Autodesk Fusion 360 part; units mm, degrees
(part 2 of 3)
  arc A308 (601.5, 1) -> (601, 0.5) centre (601.5, 0.5) ccw
  arc A309 (605, 0.5) -> (604.5, 1) centre (604.5, 0.5) ccw
  arc A310 (604.5, -3) -> (605, -2.5) centre (604.5, -2.5) ccw
  arc A311 (601, -2.5) -> (601.5, -3) centre (601.5, -2.5) ccw
  arc A312 (606.5, 1) -> (606, 0.5) centre (606.5, 0.5) ccw
  arc A313 (610, 0.5) -> (609.5, 1) centre (609.5, 0.5) ccw
  arc A314 (609.5, -3) -> (610, -2.5) centre (609.5, -2.5) ccw
  arc A315 (606, -2.5) -> (606.5, -3) centre (606.5, -2.5) ccw
  arc A316 (611.5, 1) -> (611, 0.5) centre (611.5, 0.5) ccw
  arc A317 (615, 0.5) -> (614.5, 1) centre (614.5, 0.5) ccw
  arc A318 (611, -2.5) -> (611.5, -3) centre (611.5, -2.5) ccw
  arc A319 (614.5, -3) -> (615, -2.5) centre (614.5, -2.5) ccw
  arc A320 (616.5, 1) -> (616, 0.5) centre (616.5, 0.5) ccw
  arc A321 (620, 0.5) -> (619.5, 1) centre (619.5, 0.5) ccw
  arc A322 (619.5, -3) -> (620, -2.5) centre (619.5, -2.5) ccw
  arc A323 (616, -2.5) -> (616.5, -3) centre (616.5, -2.5) ccw
  arc A324 (621, -2.5) -> (621.5, -3) centre (621.5, -2.5) ccw
  arc A325 (624.5, -3) -> (625, -2.5) centre (624.5, -2.5) ccw
  arc A326 (625, 0.5) -> (624.5, 1) centre (624.5, 0.5) ccw
  arc A327 (621.5, 1) -> (621, 0.5) centre (621.5, 0.5) ccw
  arc A328 (626.5, 1) -> (626, 0.5) centre (626.5, 0.5) ccw
  arc A329 (630, 0.5) -> (629.5, 1) centre (629.5, 0.5) ccw
  arc A330 (629.5, -3) -> (630, -2.5) centre (629.5, -2.5) ccw
  arc A331 (626, -2.5) -> (626.5, -3) centre (626.5, -2.5) ccw
  arc A332 (631, -2.5) -> (631.5, -3) centre (631.5, -2.5) ccw
  arc A333 (634.5, -3) -> (635, -2.5) centre (634.5, -2.5) ccw
  arc A334 (635, 0.5) -> (634.5, 1) centre (634.5, 0.5) ccw
  arc A335 (631.5, 1) -> (631, 0.5) centre (631.5, 0.5) ccw
  arc A336 (636.5, 1) -> (636, 0.5) centre (636.5, 0.5) ccw
  arc A337 (640, 0.5) -> (639.5, 1) centre (639.5, 0.5) ccw
  arc A338 (639.5, -3) -> (640, -2.5) centre (639.5, -2.5) ccw
  arc A339 (636, -2.5) -> (636.5, -3) centre (636.5, -2.5) ccw
  arc A340 (641.5, 1) -> (641, 0.5) centre (641.5, 0.5) ccw
  arc A341 (645, 0.5) -> (644.5, 1) centre (644.5, 0.5) ccw
  arc A342 (644.5, -3) -> (645, -2.5) centre (644.5, -2.5) ccw
  arc A343 (641, -2.5) -> (641.5, -3) centre (641.5, -2.5) ccw
  arc A344 (646.5, 1) -> (646, 0.5) centre (646.5, 0.5) ccw
  arc A345 (650, 0.5) -> (649.5, 1) centre (649.5, 0.5) ccw
  arc A346 (649.5, -3) -> (650, -2.5) centre (649.5, -2.5) ccw
  arc A347 (646, -2.5) -> (646.5, -3) centre (646.5, -2.5) ccw
  arc A348 (651.5, 1) -> (651, 0.5) centre (651.5, 0.5) ccw
  arc A349 (655, 0.5) -> (654.5, 1) centre (654.5, 0.5) ccw
  arc A350 (651, -2.5) -> (651.5, -3) centre (651.5, -2.5) ccw
  arc A351 (654.5, -3) -> (655, -2.5) centre (654.5, -2.5) ccw
  arc A352 (656.5, 1) -> (656, 0.5) centre (656.5, 0.5) ccw
  arc A353 (656, -2.5) -> (656.5, -3) centre (656.5, -2.5) ccw
  arc A354 (659.5, -3) -> (660, -2.5) centre (659.5, -2.5) ccw
  arc A355 (660, 0.5) -> (659.5, 1) centre (659.5, 0.5) ccw
  arc A356 (597.5, -4) -> (597, -4.5) centre (597.5, -4.5) ccw
  arc A357 (597, -7.5) -> (597.5, -8) centre (597.5, -7.5) ccw
  arc A358 (602.5, -8) -> (603, -7.5) centre (602.5, -7.5) ccw
  arc A359 (603, -4.5) -> (602.5, -4) centre (602.5, -4.5) ccw
  arc A360 (604.5, -4) -> (604, -4.5) centre (604.5, -4.5) ccw
  arc A361 (604, -7.5) -> (604.5, -8) centre (604.5, -7.5) ccw
  arc A362 (607.5, -8) -> (608, -7.5) centre (607.5, -7.5) ccw
  arc A363 (608, -4.5) -> (607.5, -4) centre (607.5, -4.5) ccw
  arc A364 (609.5, -4) -> (609, -4.5) centre (609.5, -4.5) ccw
  arc A365 (609, -7.5) -> (609.5, -8) centre (609.5, -7.5) ccw
  arc A366 (612.5, -8) -> (613, -7.5) centre (612.5, -7.5) ccw
  arc A367 (613, -4.5) -> (612.5, -4) centre (612.5, -4.5) ccw
  arc A368 (614.5, -4) -> (614, -4.5) centre (614.5, -4.5) ccw
  arc A369 (614, -7.5) -> (614.5, -8) centre (614.5, -7.5) ccw
  arc A370 (617.5, -8) -> (618, -7.5) centre (617.5, -7.5) ccw
  arc A371 (618, -4.5) -> (617.5, -4) centre (617.5, -4.5) ccw
  arc A372 (619.5, -4) -> (619, -4.5) centre (619.5, -4.5) ccw
  arc A373 (619, -7.5) -> (619.5, -8) centre (619.5, -7.5) ccw
  arc A374 (622.5, -8) -> (623, -7.5) centre (622.5, -7.5) ccw
  arc A375 (623, -4.5) -> (622.5, -4) centre (622.5, -4.5) ccw
  arc A376 (624.5, -4) -> (624, -4.5) centre (624.5, -4.5) ccw
  arc A377 (624, -7.5) -> (624.5, -8) centre (624.5, -7.5) ccw
  arc A378 (627.5, -8) -> (628, -7.5) centre (627.5, -7.5) ccw
  arc A379 (628, -4.5) -> (627.5, -4) centre (627.5, -4.5) ccw
  arc A380 (629.5, -4) -> (629, -4.5) centre (629.5, -4.5) ccw
  arc A381 (629, -7.5) -> (629.5, -8) centre (629.5, -7.5) ccw
  arc A382 (632.5, -8) -> (633, -7.5) centre (632.5, -7.5) ccw
  arc A383 (633, -4.5) -> (632.5, -4) centre (632.5, -4.5) ccw
  arc A384 (634.5, -4) -> (634, -4.5) centre (634.5, -4.5) ccw
  arc A385 (634, -7.5) -> (634.5, -8) centre (634.5, -7.5) ccw
  arc A386 (637.5, -8) -> (638, -7.5) centre (637.5, -7.5) ccw
  arc A387 (638, -4.5) -> (637.5, -4) centre (637.5, -4.5) ccw
  arc A388 (639.5, -4) -> (639, -4.5) centre (639.5, -4.5) ccw
  arc A389 (639, -7.5) -> (639.5, -8) centre (639.5, -7.5) ccw
  arc A390 (642.5, -8) -> (643, -7.5) centre (642.5, -7.5) ccw
  arc A391 (643, -4.5) -> (642.5, -4) centre (642.5, -4.5) ccw
  arc A392 (644.5, -4) -> (644, -4.5) centre (644.5, -4.5) ccw
  arc A393 (644, -7.5) -> (644.5, -8) centre (644.5, -7.5) ccw
  arc A394 (647.5, -8) -> (648, -7.5) centre (647.5, -7.5) ccw
  arc A395 (648, -4.5) -> (647.5, -4) centre (647.5, -4.5) ccw
  arc A396 (649.5, -4) -> (649, -4.5) centre (649.5, -4.5) ccw
  arc A397 (649, -7.5) -> (649.5, -8) centre (649.5, -7.5) ccw
  arc A398 (652.5, -8) -> (653, -7.5) centre (652.5, -7.5) ccw
  arc A399 (653, -4.5) -> (652.5, -4) centre (652.5, -4.5) ccw
  arc A400 (654.5, -4) -> (654, -4.5) centre (654.5, -4.5) ccw
  arc A401 (654, -7.5) -> (654.5, -8) centre (654.5, -7.5) ccw
  arc A402 (657.5, -8) -> (658, -7.5) centre (657.5, -7.5) ccw
  arc A403 (658, -4.5) -> (657.5, -4) centre (657.5, -4.5) ccw
  arc A404 (626, -12.5) -> (626.5, -13) centre (626.5, -12.5) ccw
  arc A405 (629.5, -13) -> (630, -12.5) centre (629.5, -12.5) ccw
  arc A406 (629, -14.5) -> (628.5, -14) centre (628.5, -14.5) ccw
  arc A407 (625.5, -14) -> (625, -14.5) centre (625.5, -14.5) ccw
  arc A408 (625, -17.5) -> (625.5, -18) centre (625.5, -17.5) ccw
  arc A409 (623.5, -18) -> (624, -17.5) centre (623.5, -17.5) ccw
  arc A410 (624, -14.5) -> (623.5, -14) centre (623.5, -14.5) ccw
  arc A411 (620.5, -14) -> (620, -14.5) centre (620.5, -14.5) ccw
  arc A412 (620, -17.5) -> (620.5, -18) centre (620.5, -17.5) ccw
  arc A413 (617.5, -19) -> (617, -19.5) centre (617.5, -19.5) ccw
  arc A414 (617, -22.5) -> (617.5, -23) centre (617.5, -22.5) ccw
  arc A415 (615.5, -23) -> (616, -22.5) centre (615.5, -22.5) ccw
  arc A416 (616, -19.5) -> (615.5, -19) centre (615.5, -19.5) ccw
  arc A417 (612.5, -19) -> (612, -19.5) centre (612.5, -19.5) ccw
  arc A418 (612, -22.5) -> (612.5, -23) centre (612.5, -22.5) ccw
  arc A419 (610.5, -23) -> (611, -22.5) centre (610.5, -22.5) ccw
  arc A420 (611, -19.5) -> (610.5, -19) centre (610.5, -19.5) ccw
  arc A421 (607.5, -19) -> (607, -19.5) centre (607.5, -19.5) ccw
  arc A422 (607, -22.5) -> (607.5, -23) centre (607.5, -22.5) ccw
  arc A423 (619, -14.5) -> (618.5, -14) centre (618.5, -14.5) ccw
  arc A424 (618.5, -18) -> (619, -17.5) centre (618.5, -17.5) ccw
  arc A425 (615, -17.5) -> (615.5, -18) centre (615.5, -17.5) ccw
  arc A426 (615.5, -14) -> (615, -14.5) centre (615.5, -14.5) ccw
  arc A427 (624.5, -13) -> (625, -12.5) centre (624.5, -12.5) ccw
  arc A428 (621.5, -9) -> (621, -9.5) centre (621.5, -9.5) ccw
  arc A429 (621, -12.5) -> (621.5, -13) centre (621.5, -12.5) ccw
  arc A430 (619.5, -13) -> (620, -12.5) centre (619.5, -12.5) ccw
  arc A431 (620, -9.5) -> (619.5, -9) centre (619.5, -9.5) ccw
  arc A432 (616.5, -9) -> (616, -9.5) centre (616.5, -9.5) ccw
  arc A433 (616, -12.5) -> (616.5, -13) centre (616.5, -12.5) ccw
  arc A434 (614.5, -13) -> (615, -12.5) centre (614.5, -12.5) ccw
  arc A435 (615, -9.5) -> (614.5, -9) centre (614.5, -9.5) ccw
  arc A436 (611.5, -9) -> (611, -9.5) centre (611.5, -9.5) ccw
  arc A437 (611, -12.5) -> (611.5, -13) centre (611.5, -12.5) ccw
  arc A438 (614, -14.5) -> (613.5, -14) centre (613.5, -14.5) ccw
  arc A439 (613.5, -18) -> (614, -17.5) centre (613.5, -17.5) ccw
  arc A440 (610, -17.5) -> (610.5, -18) centre (610.5, -17.5) ccw
  arc A441 (610.5, -14) -> (610, -14.5) centre (610.5, -14.5) ccw
  arc A442 (609.5, -13) -> (610, -12.5) centre (609.5, -12.5) ccw
  arc A443 (610, -9.5) -> (609.5, -9) centre (609.5, -9.5) ccw
  arc A444 (606.5, -9) -> (606, -9.5) centre (606.5, -9.5) ccw
  arc A445 (606, -12.5) -> (606.5, -13) centre (606.5, -12.5) ccw
  arc A446 (609, -14.5) -> (608.5, -14) centre (608.5, -14.5) ccw
  arc A447 (608.5, -18) -> (609, -17.5) centre (608.5, -17.5) ccw
  arc A448 (606, -19.5) -> (605.5, -19) centre (605.5, -19.5) ccw
  arc A449 (605.5, -23) -> (606, -22.5) centre (605.5, -22.5) ccw
  arc A450 (597.5, -9) -> (597, -9.5) centre (597.5, -9.5) ccw
  arc A451 (605, -9.5) -> (604.5, -9) centre (604.5, -9.5) ccw
  arc A452 (597, -12.5) -> (597.5, -13) centre (597.5, -12.5) ccw
  arc A453 (604.5, -13) -> (605, -12.5) centre (604.5, -12.5) ccw
  arc A454 (597.5, -14) -> (597, -14.5) centre (597.5, -14.5) ccw
  arc A455 (597, -17.5) -> (597.5, -18) centre (597.5, -17.5) ccw
  arc A456 (597.5, -19) -> (597, -19.5) centre (597.5, -19.5) ccw
  arc A457 (601, -19.5) -> (600.5, -19) centre (600.5, -19.5) ccw
  arc A458 (600.5, -23) -> (601, -22.5) centre (600.5, -22.5) ccw
  arc A459 (597, -22.5) -> (597.5, -23) centre (597.5, -22.5) ccw
  arc A460 (602, -22.5) -> (602.5, -23) centre (602.5, -22.5) ccw
  arc A461 (602.5, -19) -> (602, -19.5) centre (602.5, -19.5) ccw
  arc A462 (616.5, -25) -> (615, -26.5) centre (616.5, -26.5) ccw
  arc A463 (643, -27) -> (641, -25) centre (641, -27) ccw
  arc A464 (641, -47) -> (643, -45) centre (641, -45) ccw
  arc A465 (615, -45) -> (617, -47) centre (617, -45) ccw
  arc A466 (695, 8) -> (693, 10) centre (693, 8) ccw
  arc A467 (592, 10) -> (590, 8) centre (592, 8) ccw
  arc A468 (590, -53) -> (592, -55) centre (592, -53) ccw
  arc A469 (693, -55) -> (695, -53) centre (693, -53) ccw
  arc A470 (693, 20) -> (695, 22) centre (693, 22) ccw
  arc A471 (691, 24) -> (693, 26) centre (691, 26) ccw
  arc A472 (590, 22) -> (592, 20) centre (592, 22) ccw
  arc A473 (592, 26) -> (594, 24) centre (594, 26) ccw
  arc A474 (693, 80) -> (691, 82) centre (691, 80) ccw
  arc A475 (695, 83) -> (693, 85) centre (693, 83) ccw
  arc A476 (594, 82) -> (592, 80) centre (594, 80) ccw
  arc A477 (592, 85) -> (590, 83) centre (592, 83) ccw
  dimension "d35" = 160
  dimension "d36" = 8
  dimension "d37" = 8
  dimension "d38" = 8
  dimension "d40" = 8
  dimension "d41" = 8
  dimension "d42" = 20
  dimension "d43" = 165
  dimension "d44" = 70
  dimension "d45" = 32
  dimension "d46" = 24
  dimension "d47" = 108
  dimension "d48" = 40
  dimension "d49" = 60
  dimension "d50" = 48
  dimension "d51" = 15
  dimension "d52" = 28
  dimension "d53" = 48
  dimension "d54" = 15
  dimension "d55" = 28
  dimension "d59" = 20
  dimension "d60" = 40
  dimension "d61" = 70
  dimension "d62" = 20
  dimension "d63" = 60
  dimension "d64" = 18
  dimension "d65" = 18
  dimension "d66" = 5
  dimension "d67" = 19
  dimension "d68" = 19
  dimension "d69" = 150
  dimension "d70" = 180
  dimension "d72" = 15
  dimension "d73" = 328
  dimension "d74" = 60
  dimension "d75" = 90
  dimension "d77" = 360
  dimension "d144" = 1
  dimension "d146" = 1
  dimension "d147" = 0
  dimension "d148" = 1
  dimension "d149" = 0
  dimension "d150" = 1
  dimension "d151" = 0
  dimension "d152" = 1
  dimension "d153" = 0
  dimension "d154" = 1
  dimension "d155" = 0
  dimension "d156" = 1
  dimension "d157" = 0
  dimension "d158" = 1
  dimension "d159" = 0
  dimension "d160" = 1
  dimension "d161" = 0
  dimension "d162" = 1
  dimension "d163" = 0
  dimension "d164" = 1
  dimension "d165" = 0
  dimension "d166" = 1
  dimension "d167" = 0
  dimension "d168" = 1
  dimension "d169" = 0
  dimension "d172" = 0.7
  dimension "d174" = 0.7
  dimension "d176" = 0.5
  dimension "d177" = 0.5
  dimension "d178" = 1.5
  dimension "d179" = 2
  constraint horizontal L0
  constraint vertical L1
  constraint horizontal L2
  constraint vertical L3
  constraint tangent L1 A0
  constraint tangent L2 A0
  constraint tangent L2 A1
  constraint tangent L3 A1
  constraint concentric A2 A3
  constraint coincident A2.centre A3.centre
  constraint perpendicular L4 L5
  constraint coincident L5.end A4.centre
  constraint concentric A4 A5
  constraint coincident A5 L6.start
  constraint tangent A5 L6
  constraint perpendicular L2 L6
  constraint perpendicular L6 L7
  constraint tangent A5 L8
  constraint coincident L2 A1.start
  constraint tangent L8 A6
  constraint tangent L2 A6
  constraint tangent A3 A7
  constraint tangent A5 A7
  constraint coincident A5 A7.end
  constraint coincident A3 A7.start
  constraint coincident A5 L9.start
  constraint parallel L8 L9
  constraint perpendicular L4 L10
  constraint coincident L10 L11.end
  constraint perpendicular L9 L12
  constraint tangent A3 A8
  constraint coincident L2 L15.end
  constraint tangent L15 A8
  constraint coincident A3 A8.start
  constraint tangent L14 A9
  constraint tangent A8 A9
  constraint tangent L13 A10
  constraint tangent L14 A10
  constraint tangent L9 A11
  constraint tangent L12 A11
  constraint tangent L13 A12
  constraint tangent A3 A12
  constraint coincident A3 A12.end
  constraint tangent L12 A13
  constraint tangent A3 A13
  constraint coincident A3 A13.start
  constraint tangent L15 A14
  constraint tangent A8 A14
  constraint coincident A8 A14.end
  constraint coincident L15 A14.start
  constraint concentric A18 A28
  constraint coincident L16.end A15.centre
  constraint concentric A15 A19
  constraint perpendicular L16 L17
  constraint coincident L17.end A20.centre
  constraint concentric A20 A21
  constraint parallel L17 L18
  constraint parallel L16 L19
  constraint tangent L19 A16
  constraint tangent L18 A16
  constraint tangent A17 A19
  constraint parallel L17 L20
  constraint coincident L20 A18.end
  constraint concentric A28 A29
  constraint coincident L16.start L17.start
  constraint coincident A18.centre L21.start
  constraint coincident A24.centre A29
  constraint coincident L21 A24.centre
  constraint coincident A25.centre A29
  constraint coincident L22 A25.centre
  constraint tangent A22 A25
  constraint coincident L22 A22.end
  constraint coincident L21 A22.start
  constraint tangent A23 A25
  constraint coincident L22 A23.end
  constraint coincident L21 A23.start
  constraint coincident L23.start A27
  constraint coincident L16 L23.start
  constraint tangent L23 A27
  constraint tangent L23 A26
  constraint tangent A26 A28
  constraint coincident L20 A27.end
  constraint coincident L17 A27.start
  constraint coincident L20 A28.end
  constraint coincident L20 A29.end
  constraint coincident L20 A29.start
  constraint symmetric A15 L20 A34
  constraint symmetric L18.start L20 L24.start
  constraint symmetric L19.start L20 L25.start
  constraint symmetric L19.end L20 A32.end
  constraint symmetric L18.end L20 L24.end
  constraint symmetric A16 L20 A32
  constraint symmetric A17.end L20 A33.start
  constraint symmetric A17 L20 A36
  constraint symmetric A18 L20 A37
  constraint symmetric A19 L20 A33
  constraint symmetric A20 L20 A31
  constraint symmetric A20.start L20 A31.end
  constraint symmetric A21.end L20 A30.start
  constraint symmetric A21.start L20 A30.end
  constraint symmetric A21 L20 A30
  constraint symmetric L20 A18.end A37.start
  constraint symmetric L20 A22.start A39.end
  constraint symmetric L20 A22.end A39.start
  constraint symmetric L20 A22 A39
  constraint symmetric L20 A23.start A38.end
  constraint symmetric L20 A23.end A38.start
  constraint symmetric L20 A23 A38
  constraint symmetric L20 A24 A41
  constraint symmetric L20 A25 A40
  constraint symmetric L20 L23.start L26.start
  constraint symmetric L20 L23.end L26.end
  constraint symmetric L20 A26 A43
  constraint symmetric L20 A26.start A42.end
  constraint symmetric L20 A27.end A35.start
  constraint symmetric L20 A27.start A35.end
  constraint symmetric L20 A27 A35
  constraint symmetric L20 A28.end A42.start
  constraint symmetric L20 A28 A42
  constraint coincident A18 L22.end
  constraint tangent A36 A44
  constraint tangent A37 A44
  constraint tangent A17 A45
  constraint tangent A18 A45
  constraint concentric A46 A47
  constraint vertical L27
  constraint parallel L27 L28
  constraint coincident A47 L28.end
  constraint symmetric L27 L28.end L29.end
  constraint concentric A47 A50
  constraint coincident A48.centre A50
  constraint coincident L27 A48.centre
  constraint concentric A48 A49
  constraint coincident A49 L29.start
  constraint coincident A49 L28.start
  constraint horizontal L40
  constraint vertical L41
  constraint horizontal L42
  constraint vertical L43
  constraint horizontal L44
  constraint vertical L45
  constraint horizontal L46
  constraint vertical L47
  constraint horizontal L48
  constraint vertical L49
  constraint horizontal L50
  constraint vertical L51
  constraint horizontal L52
  constraint vertical L53
  constraint horizontal L54
  constraint vertical L55
  constraint horizontal L104
  constraint vertical L105
  constraint horizontal L106
  constraint vertical L107
  constraint horizontal L148
  constraint vertical L149
  constraint horizontal L150
  constraint vertical L151
  constraint horizontal L152
  constraint vertical L153
  constraint horizontal L154
  constraint vertical L155
  constraint horizontal L192
  constraint vertical L193
  constraint horizontal L194
  constraint vertical L195
  constraint horizontal L196
  constraint vertical L197
  constraint horizontal L198
  constraint vertical L199
  constraint horizontal L200
  constraint vertical L201
  constraint horizontal L202
  constraint vertical L203
  constraint horizontal L248
  constraint vertical L249
  constraint horizontal L250
  constraint vertical L251
  constraint horizontal L252
  constraint vertical L253
  constraint horizontal L254
  constraint vertical L255
  constraint horizontal L324
  constraint vertical L325
  constraint horizontal L326
  constraint vertical L327
  constraint horizontal L328
  constraint vertical L329
  constraint horizontal L330
  constraint vertical L331
  constraint horizontal L332
  constraint vertical L333
  constraint horizontal L334
  constraint vertical L335
  constraint horizontal L336
  constraint vertical L337
  constraint horizontal L338
  constraint vertical L339
  constraint horizontal L340
  constraint vertical L341
  constraint horizontal L342
  constraint vertical L343
  constraint horizontal L383
  constraint horizontal L388
  constraint vertical L389
  constraint horizontal L390
  constraint vertical L391
  constraint horizontal L392
  constraint vertical L393
  constraint horizontal L394
  constraint vertical L395
  constraint horizontal L396
  constraint vertical L397
  constraint horizontal L398
  constraint vertical L399
  constraint horizontal L400
  constraint vertical L401
  constraint horizontal L402
  constraint vertical L403
  constraint horizontal L404
  constraint vertical L405
  constraint horizontal L406
  constraint vertical L407
  constraint horizontal L408
  constraint vertical L409
  constraint horizontal L410
  constraint vertical L411
  constraint horizontal L412
  constraint vertical L413
  constraint horizontal L414
  constraint vertical L415
  constraint horizontal L416
  constraint vertical L417
  constraint horizontal L418
  constraint vertical L419
  constraint horizontal L420
  constraint vertical L421
  constraint horizontal L422
  constraint vertical L423
  constraint horizontal L424
  constraint vertical L425
  constraint horizontal L426
  constraint vertical L427
  constraint horizontal L428
  constraint vertical L429
  constraint horizontal L430
  constraint vertical L431
  constraint horizontal L432
  constraint vertical L433
  constraint horizontal L434
  constraint vertical L435
  constraint horizontal L436
  constraint vertical L437
  constraint horizontal L438
  constraint vertical L439
  constraint horizontal L440
  constraint vertical L441
  constraint horizontal L442
  constraint vertical L443
  constraint perpendicular L443 L444
  constraint horizontal L449
  constraint vertical L450
  constraint horizontal L451
  constraint vertical L452
  constraint tangent L254 A69
  constraint tangent L255 A69
  constraint tangent L253 A70
  constraint tangent L254 A70
  constraint equal A69 A70
  constraint tangent L252 A71
  constraint tangent L253 A71
  constraint equal A69 A71
  constraint tangent L252 A72
  constraint tangent L255 A72
  constraint equal A69 A72
  constraint tangent L258 A73
  constraint tangent L259 A73
  constraint equal A69 A73
  constraint tangent L256 A74
  constraint tangent L258 A74
  constraint equal A69 A74
  constraint tangent L256 A75
  constraint tangent L257 A75
  constraint equal A69 A75
  constraint tangent L257 A76
  constraint tangent L259 A76
  constraint equal A69 A76
  constraint tangent L262 A77
  constraint tangent L263 A77
  constraint equal A69 A77
  constraint tangent L260 A78
  constraint tangent L262 A78
  constraint equal A69 A78
  constraint tangent L261 A79
  constraint tangent L263 A79
  constraint equal A69 A79
  constraint tangent L260 A80
  constraint tangent L261 A80
  constraint equal A69 A80
  constraint tangent L266 A81
  constraint tangent L267 A81
  constraint equal A69 A81
  constraint tangent L264 A82
  constraint tangent L266 A82
  constraint equal A69 A82
  constraint tangent L264 A83
  constraint tangent L265 A83
  constraint equal A69 A83
  constraint tangent L265 A84
  constraint tangent L267 A84
  constraint equal A69 A84
  constraint tangent L268 A85
  constraint tangent L270 A85
  constraint equal A69 A85
  constraint tangent L270 A86
  constraint tangent L271 A86
  constraint equal A69 A86
  constraint tangent L269 A87
  constraint tangent L271 A87
  constraint equal A69 A87
  constraint tangent L268 A88
  constraint tangent L269 A88
  constraint equal A69 A88
  constraint tangent L272 A89
  constraint tangent L274 A89
  constraint equal A69 A89
  constraint tangent L274 A90
  constraint tangent L275 A90
  constraint equal A69 A90
  constraint tangent L273 A91
  constraint tangent L275 A91
  constraint equal A69 A91
  constraint tangent L272 A92
  constraint tangent L273 A92
  constraint equal A69 A92
  constraint tangent L276 A93
  constraint tangent L278 A93
  constraint equal A69 A93
  constraint tangent L278 A94
  constraint tangent L279 A94
  constraint equal A69 A94
  constraint tangent L277 A95
  constraint tangent L279 A95
  constraint equal A69 A95
  constraint tangent L276 A96
  constraint tangent L277 A96
  constraint equal A69 A96
  constraint tangent L280 A97
  constraint tangent L282 A97
  constraint equal A69 A97
  constraint tangent L282 A98
  constraint tangent L283 A98
  constraint equal A69 A98
  constraint tangent L281 A99
  constraint tangent L283 A99
  constraint equal A69 A99
  constraint tangent L280 A100
  constraint tangent L281 A100
  constraint equal A69 A100
  constraint tangent L284 A101
  constraint tangent L286 A101
  constraint equal A69 A101
  constraint tangent L284 A102
  constraint tangent L285 A102
  constraint equal A69 A102
  constraint tangent L285 A103
  constraint tangent L287 A103
  constraint equal A69 A103
  constraint tangent L286 A104
  constraint tangent L287 A104
  constraint equal A69 A104
  constraint tangent L288 A105
  constraint tangent L290 A105
  constraint equal A69 A105
  constraint tangent L288 A106
  constraint tangent L289 A106
  constraint equal A69 A106
  constraint tangent L289 A107
  constraint tangent L291 A107
  constraint equal A69 A107
  constraint tangent L290 A108
  constraint tangent L291 A108
  constraint equal A69 A108
  constraint tangent L292 A109
  constraint tangent L294 A109
  constraint equal A69 A109
  constraint tangent L292 A110
  constraint tangent L293 A110
  constraint equal A69 A110
  constraint tangent L293 A111
  constraint tangent L295 A111
  constraint equal A69 A111
  constraint tangent L294 A112
  constraint tangent L295 A112
  constraint equal A69 A112
  constraint tangent L298 A113
  constraint tangent L299 A113
  constraint equal A69 A113
  constraint tangent L297 A114
  constraint tangent L299 A114
  constraint equal A69 A114
  constraint tangent L296 A115
  constraint tangent L297 A115
  constraint equal A69 A115
  constraint tangent L296 A116
  constraint tangent L298 A116
  constraint equal A69 A116
  constraint tangent L300 A117
  constraint tangent L302 A117
  constraint equal A69 A117
  constraint tangent L300 A118
  constraint tangent L301 A118
  constraint equal A69 A118
  constraint tangent L301 A119
  constraint tangent L303 A119
  constraint equal A69 A119
  constraint tangent L302 A120
  constraint tangent L303 A120
  constraint equal A69 A120
  constraint tangent L306 A121
  constraint tangent L307 A121
  constraint equal A69 A121
  constraint tangent L305 A122
  constraint tangent L307 A122
  constraint equal A69 A122
  constraint tangent L304 A123
  constraint tangent L305 A123
  constraint equal A69 A123
  constraint tangent L304 A124
  constraint tangent L306 A124
  constraint equal A69 A124
  constraint tangent L308 A125
  constraint tangent L310 A125
  constraint equal A69 A125
  constraint tangent L308 A126
  constraint tangent L309 A126
  constraint equal A69 A126
  constraint tangent L309 A127
  constraint tangent L311 A127
  constraint equal A69 A127
  constraint tangent L311 A128
  constraint tangent L310 A128
  constraint equal A69 A128
  constraint tangent L314 A129
  constraint tangent L315 A129
  constraint equal A69 A129
  constraint tangent L314 A130
  constraint tangent L312 A130
  constraint equal A69 A130
  constraint tangent L312 A131
  constraint tangent L313 A131
  constraint equal A69 A131
  constraint tangent L313 A132
  constraint tangent L315 A132
  constraint equal A69 A132
  constraint tangent L318 A133
  constraint tangent L319 A133
  constraint equal A69 A133
  constraint tangent L316 A134
  constraint tangent L318 A134
  constraint equal A69 A134
  constraint tangent L316 A135
  constraint tangent L317 A135
  constraint equal A69 A135
  constraint tangent L317 A136
  constraint tangent L319 A136
  constraint equal A69 A136
  constraint tangent L322 A137
  constraint tangent L323 A137
  constraint equal A69 A137
  constraint tangent L320 A138
  constraint tangent L322 A138
  constraint equal A69 A138
  constraint tangent L321 A139
  constraint tangent L323 A139
  constraint equal A69 A139
  constraint tangent L320 A140
  constraint tangent L321 A140
  constraint equal A69 A140
  constraint tangent L336 A141
  constraint tangent L337 A141
  constraint equal A69 A141
  constraint tangent L337 A142
  constraint tangent L338 A142
  constraint equal A69 A142
  constraint tangent L338 A143
  constraint tangent L339 A143
  constraint equal A69 A143
  constraint tangent L336 A144
  constraint tangent L339 A144
  constraint equal A69 A144
  constraint tangent L333 A145
  constraint tangent L334 A145
  constraint equal A69 A145
  constraint tangent L334 A146
  constraint tangent L335 A146
  constraint equal A69 A146
  constraint tangent L332 A147
  constraint tangent L335 A147
  constraint equal A69 A147
  constraint tangent L332 A148
  constraint tangent L333 A148
  constraint equal A69 A148
  constraint tangent L329 A149
  constraint tangent L330 A149
  constraint equal A69 A149
  constraint tangent L330 A150
  constraint tangent L331 A150
  constraint equal A69 A150
  constraint tangent L328 A151
  constraint tangent L331 A151
  constraint equal A69 A151
  constraint tangent L328 A152
  constraint tangent L329 A152
  constraint equal A69 A152
  constraint tangent L325 A153
  constraint tangent L326 A153
  constraint equal A69 A153
  constraint tangent L326 A154
  constraint tangent L327 A154
  constraint equal A69 A154
  constraint tangent L324 A155
  constraint tangent L325 A155
  constraint equal A69 A155
  constraint tangent L324 A156
  constraint tangent L327 A156
  constraint equal A69 A156
  constraint tangent L248 A157
  constraint tangent L249 A157
  constraint equal A69 A157
  constraint tangent L248 A158
  constraint tangent L251 A158
  constraint equal A69 A158
  constraint tangent L250 A159
  constraint tangent L251 A159
  constraint equal A69 A159
  constraint tangent L249 A160
  constraint tangent L250 A160
  constraint equal A69 A160
  constraint tangent L352 A161
  constraint tangent L367 A161
  constraint equal A69 A161
  constraint tangent L352 A162
  constraint tangent L366 A162
  constraint equal A69 A162
  constraint tangent L365 A163
  constraint tangent L366 A163
  constraint equal A69 A163
  constraint tangent L365 A164
  constraint tangent L367 A164
  constraint equal A69 A164
  constraint tangent L350 A165
  constraint tangent L351 A165
  constraint equal A69 A165
  constraint tangent L348 A166
  constraint tangent L350 A166
  constraint equal A69 A166
  constraint tangent L348 A167
  constraint tangent L349 A167
  constraint equal A69 A167
  constraint tangent L349 A168
  constraint tangent L351 A168
  constraint equal A69 A168
  constraint tangent L346 A169
  constraint tangent L347 A169
  constraint equal A69 A169
  constraint tangent L344 A170
  constraint tangent L346 A170
  constraint equal A69 A170
  constraint tangent L344 A171
  constraint tangent L345 A171
  constraint equal A69 A171
  constraint tangent L345 A172
  constraint tangent L347 A172
  constraint equal A69 A172
  constraint tangent L359 A173
  constraint tangent L360 A173
  constraint equal A69 A173
  constraint tangent L357 A174
  constraint tangent L359 A174
  constraint equal A69 A174
  constraint tangent L362 A175
  constraint tangent L364 A175
  constraint equal A69 A175
  constraint tangent L363 A176
  constraint tangent L364 A176
  constraint equal A69 A176
  constraint tangent L361 A177
  constraint tangent L362 A177
  constraint equal A69 A177
  constraint tangent L388 A178
  constraint tangent L391 A178
  constraint equal A69 A178
  constraint tangent L388 A179
  constraint tangent L389 A179
  constraint equal A69 A179
  constraint tangent L389 A180
  constraint tangent L390 A180
  constraint equal A69 A180
  constraint tangent L390 A181
  constraint tangent L391 A181
  constraint equal A69 A181
  constraint tangent L384 A182
  constraint tangent L386 A182
  constraint equal A69 A182
  constraint tangent L386 A183
  constraint tangent L387 A183
  constraint equal A69 A183
  constraint tangent L385 A184
  constraint tangent L387 A184
  constraint equal A69 A184
  constraint tangent L384 A185
  constraint tangent L385 A185
  constraint equal A69 A185
  constraint tangent L376 A186
  constraint tangent L378 A186
  constraint equal A69 A186
  constraint tangent L378 A187
  constraint tangent L379 A187
  constraint equal A69 A187
  constraint tangent L377 A188
  constraint tangent L379 A188
  constraint equal A69 A188
  constraint tangent L376 A189
  constraint tangent L377 A189
  constraint equal A69 A189
  constraint tangent L372 A190
  constraint tangent L374 A190
  constraint equal A69 A190
  constraint tangent L374 A191
  constraint tangent L375 A191
  constraint equal A69 A191
  constraint tangent L373 A192
  constraint tangent L375 A192
  constraint equal A69 A192
  constraint tangent L372 A193
  constraint tangent L373 A193
  constraint equal A69 A193
  constraint tangent L382 A194
  constraint tangent L383 A194
  constraint equal A69 A194
  constraint tangent L382 A195
  constraint tangent L380 A195
  constraint equal A69 A195
  constraint tangent L380 A196
  constraint tangent L381 A196
  constraint equal A69 A196
  constraint tangent L381 A197
  constraint tangent L383 A197
  constraint equal A69 A197
  constraint tangent L368 A198
  constraint tangent L370 A198
  constraint equal A69 A198
  constraint tangent L370 A199
  constraint tangent L371 A199
  constraint equal A69 A199
  constraint tangent L369 A200
  constraint tangent L371 A200
  constraint equal A69 A200
  constraint tangent L368 A201
  constraint tangent L369 A201
  constraint equal A69 A201
  constraint tangent L357 A202
  constraint tangent L358 A202
  constraint equal A69 A202
  constraint tangent L358 A203
  constraint tangent L360 A203
  constraint equal A69 A203
  constraint tangent L355 A204
  constraint tangent L356 A204
  constraint equal A69 A204
  constraint tangent L353 A205
  constraint tangent L355 A205
  constraint equal A69 A205
  constraint tangent L353 A206
  constraint tangent L354 A206
  constraint equal A69 A206
  constraint tangent L354 A207
  constraint tangent L356 A207
  constraint equal A69 A207
  constraint tangent L341 A208
  constraint tangent L342 A208
  constraint equal A69 A208
  constraint tangent L340 A209
  constraint tangent L341 A209
  constraint equal A69 A209
  constraint tangent L340 A210
  constraint tangent L343 A210
  constraint equal A69 A210
  constraint tangent L342 A211
  constraint tangent L343 A211
  constraint equal A69 A211
  constraint tangent L410 A212
  constraint tangent L411 A212
  constraint equal A69 A212
  constraint tangent L408 A213
  constraint tangent L411 A213
  constraint equal A69 A213
  constraint tangent L408 A214
  constraint tangent L409 A214
  constraint equal A69 A214
  constraint tangent L409 A215
  constraint tangent L410 A215
  constraint equal A69 A215
  constraint tangent L417 A216
  constraint tangent L418 A216
  constraint equal A69 A216
  constraint tangent L416 A217
  constraint tangent L417 A217
  constraint equal A69 A217
  constraint tangent L416 A218
  constraint tangent L419 A218
  constraint equal A69 A218
  constraint tangent L418 A219
  constraint tangent L419 A219
  constraint equal A69 A219
  constraint tangent L414 A220
  constraint tangent L415 A220
  constraint equal A69 A220
  constraint tangent L412 A221
  constraint tangent L415 A221
  constraint equal A69 A221
  constraint tangent L412 A222
  constraint tangent L413 A222
  constraint equal A69 A222
  constraint tangent L413 A223
  constraint tangent L414 A223
  constraint equal A69 A223
  constraint tangent L193 A224
  constraint tangent L194 A224
  constraint equal A69 A224
  constraint tangent L192 A225
  constraint tangent L193 A225
  constraint equal A69 A225
  constraint tangent L192 A226
  constraint tangent L195 A226
  constraint equal A69 A226
  constraint tangent L194 A227
  constraint tangent L195 A227
  constraint equal A69 A227
  constraint tangent L149 A228
  constraint tangent L150 A228
  constraint equal A69 A228
  constraint tangent L148 A229
  constraint tangent L149 A229
  constraint equal A69 A229
  constraint tangent L148 A230
  constraint tangent L151 A230
  constraint equal A69 A230
  constraint tangent L150 A231
  constraint tangent L151 A231
  constraint equal A69 A231
  constraint tangent L100 A232
  constraint tangent L102 A232
  constraint equal A69 A232
  constraint tangent L102 A233
  constraint tangent L103 A233
  constraint equal A69 A233
  constraint tangent L101 A234
  constraint tangent L103 A234
  constraint equal A69 A234
  constraint tangent L100 A235
  constraint tangent L101 A235
  constraint equal A69 A235
  constraint tangent L96 A236
  constraint tangent L98 A236
  constraint equal A69 A236
  constraint tangent L98 A237
  constraint tangent L99 A237
  constraint equal A69 A237
  constraint tangent L97 A238
  constraint tangent L99 A238
  constraint equal A69 A238
  constraint tangent L96 A239
  constraint tangent L97 A239
  constraint equal A69 A239
  constraint tangent L146 A240
  constraint tangent L147 A240
  constraint equal A69 A240
  constraint tangent L145 A241
  constraint tangent L146 A241
  constraint equal A69 A241
  constraint tangent L144 A242
  constraint tangent L145 A242
  constraint equal A69 A242
  constraint tangent L144 A243
  constraint tangent L147 A243
  constraint equal A69 A243
  constraint tangent L190 A244
  constraint tangent L191 A244
  constraint equal A69 A244
  constraint tangent L189 A245
  constraint tangent L190 A245
  constraint equal A69 A245
  constraint tangent L188 A246
  constraint tangent L189 A246
  constraint equal A69 A246
  constraint tangent L188 A247
  constraint tangent L191 A247
  constraint equal A69 A247
  constraint tangent L420 A248
  constraint tangent L423 A248
  constraint equal A69 A248
  constraint tangent L420 A249
  constraint tangent L421 A249
  constraint equal A69 A249
  constraint tangent L421 A250
  constraint tangent L422 A250
  constraint equal A69 A250
  constraint tangent L422 A251
  constraint tangent L423 A251
  constraint equal A69 A251
  constraint tangent L426 A252
  constraint tangent L427 A252
  constraint equal A69 A252
  constraint tangent L424 A253
  constraint tangent L427 A253
  constraint equal A69 A253
  constraint tangent L424 A254
  constraint tangent L425 A254
  constraint equal A69 A254
  constraint tangent L425 A255
  constraint tangent L426 A255
  constraint equal A69 A255
  constraint tangent L430 A256
  constraint tangent L431 A256
  constraint equal A69 A256
  constraint tangent L429 A257
  constraint tangent L430 A257
  constraint equal A69 A257
  constraint tangent L428 A258
  constraint tangent L429 A258
  constraint equal A69 A258
  constraint tangent L428 A259
  constraint tangent L431 A259
  constraint equal A69 A259
  constraint tangent L184 A260
  constraint tangent L187 A260
  constraint equal A69 A260
  constraint tangent L186 A261
  constraint tangent L187 A261
  constraint equal A69 A261
  constraint tangent L185 A262
  constraint tangent L186 A262
  constraint equal A69 A262
  constraint tangent L184 A263
  constraint tangent L185 A263
  constraint equal A69 A263
  constraint tangent L180 A264
  constraint tangent L183 A264
  constraint equal A69 A264
  constraint tangent L182 A265
  constraint tangent L183 A265
  constraint equal A69 A265
  constraint tangent L181 A266
  constraint tangent L182 A266
  constraint equal A69 A266
  constraint tangent L180 A267
  constraint tangent L181 A267
  constraint equal A69 A267
  constraint tangent L176 A268
  constraint tangent L179 A268
  constraint equal A69 A268
  constraint tangent L178 A269
  constraint tangent L179 A269
  constraint equal A69 A269
  constraint tangent L177 A270
  constraint tangent L178 A270
  constraint equal A69 A270
  constraint tangent L176 A271
  constraint tangent L177 A271
  constraint equal A69 A271
  constraint tangent L432 A272
  constraint tangent L433 A272
  constraint equal A69 A272
  constraint tangent L433 A273
  constraint tangent L434 A273
  constraint equal A69 A273
  constraint tangent L172 A274
  constraint tangent L175 A274
  constraint equal A69 A274
  constraint tangent L172 A275
  constraint tangent L173 A275
  constraint equal A69 A275
  constraint tangent L173 A276
  constraint tangent L174 A276
  constraint equal A69 A276
  constraint tangent L174 A277
  constraint tangent L175 A277
  constraint equal A69 A277
  constraint tangent L140 A278
  constraint tangent L143 A278
  constraint equal A69 A278
  constraint tangent L140 A279
  constraint tangent L141 A279
  constraint equal A69 A279
  constraint tangent L136 A280
  constraint tangent L139 A280
  constraint equal A69 A280
  constraint tangent L136 A281
  constraint tangent L137 A281
  constraint equal A69 A281
  constraint tangent L132 A282
  constraint tangent L135 A282
  constraint equal A69 A282
  constraint tangent L132 A283
  constraint tangent L133 A283
  constraint equal A69 A283
  constraint tangent L128 A284
  constraint tangent L131 A284
  constraint equal A69 A284
  constraint tangent L128 A285
  constraint tangent L129 A285
  constraint equal A69 A285
  constraint tangent L124 A286
  constraint tangent L127 A286
  constraint equal A69 A286
  constraint tangent L125 A287
  constraint tangent L124 A287
  constraint equal A69 A287
  constraint tangent L168 A288
  constraint tangent L171 A288
  constraint equal A69 A288
  constraint tangent L168 A289
  constraint tangent L169 A289
  constraint equal A69 A289
  constraint tangent L170 A290
  constraint tangent L171 A290
  constraint equal A69 A290
  constraint tangent L164 A291
  constraint tangent L167 A291
  constraint equal A69 A291
  constraint tangent L142 A292
  constraint tangent L143 A292
  constraint equal A69 A292
  constraint tangent L141 A293
  constraint tangent L142 A293
  constraint equal A69 A293
  constraint tangent L138 A294
  constraint tangent L139 A294
  constraint equal A69 A294
  constraint tangent L138 A295
  constraint tangent L137 A295
  constraint equal A69 A295
  constraint tangent L134 A296
  constraint tangent L135 A296
  constraint equal A69 A296
  constraint tangent L133 A297
  constraint tangent L134 A297
  constraint equal A69 A297
  constraint tangent L130 A298
  constraint tangent L131 A298
  constraint equal A69 A298
  constraint tangent L129 A299
  constraint tangent L130 A299
  constraint equal A69 A299
  constraint tangent L126 A300
  constraint tangent L127 A300
  constraint equal A69 A300
  constraint tangent L125 A301
  constraint tangent L126 A301
  constraint equal A69 A301
  constraint tangent L122 A302
  constraint tangent L123 A302
  constraint equal A69 A302
  constraint tangent L121 A303
  constraint tangent L122 A303
  constraint equal A69 A303
  constraint tangent L198 A304
  constraint tangent L199 A304
  constraint tangent L197 A305
  constraint tangent L198 A305
  constraint equal A304 A305
  constraint tangent L196 A306
  constraint tangent L199 A306
  constraint equal A304 A306
  constraint tangent L196 A307
  constraint tangent L197 A307
  constraint equal A304 A307
  constraint tangent L200 A308
  constraint tangent L203 A308
  constraint equal A304 A308
  constraint tangent L200 A309
  constraint tangent L201 A309
  constraint equal A304 A309
  constraint tangent L201 A310
  constraint tangent L202 A310
  constraint equal A304 A310
  constraint tangent L202 A311
  constraint tangent L203 A311
  constraint equal A304 A311
  constraint tangent L205 A312
  constraint tangent L206 A312
  constraint equal A304 A312
  constraint tangent L206 A313
  constraint tangent L207 A313
  constraint equal A304 A313
  constraint tangent L204 A314
  constraint tangent L207 A314
  constraint equal A304 A314
  constraint tangent L204 A315
  constraint tangent L205 A315
  constraint equal A304 A315
  constraint tangent L209 A316
  constraint tangent L210 A316
  constraint equal A304 A316
  constraint tangent L210 A317
  constraint tangent L211 A317
  constraint equal A304 A317
  constraint tangent L208 A318
  constraint tangent L209 A318
  constraint equal A304 A318
  constraint tangent L208 A319
  constraint tangent L211 A319
  constraint equal A304 A319
  constraint tangent L213 A320
  constraint tangent L214 A320
  constraint equal A304 A320
  constraint tangent L214 A321
  constraint tangent L215 A321
  constraint equal A304 A321
  constraint tangent L212 A322
  constraint tangent L215 A322
  constraint equal A304 A322
  constraint tangent L212 A323
  constraint tangent L213 A323
  constraint equal A304 A323
  constraint tangent L216 A324
  constraint tangent L217 A324
  constraint equal A304 A324
  constraint tangent L216 A325
  constraint tangent L219 A325
  constraint equal A304 A325
  constraint tangent L218 A326
  constraint tangent L219 A326
  constraint equal A304 A326
  constraint tangent L217 A327
  constraint tangent L218 A327
  constraint equal A304 A327
  constraint tangent L221 A328
  constraint tangent L222 A328
  constraint equal A304 A328
  constraint tangent L222 A329
  constraint tangent L223 A329
  constraint equal A304 A329
  constraint tangent L220 A330
  constraint tangent L223 A330
  constraint equal A304 A330
  constraint tangent L220 A331
  constraint tangent L221 A331
  constraint equal A304 A331
  constraint tangent L224 A332
  constraint tangent L225 A332
  constraint equal A304 A332
  constraint tangent L224 A333
  constraint tangent L227 A333
  constraint equal A304 A333
  constraint tangent L226 A334
  constraint tangent L227 A334
  constraint equal A304 A334
  constraint tangent L225 A335
  constraint tangent L226 A335
  constraint equal A304 A335
  constraint tangent L229 A336
  constraint tangent L230 A336
  constraint equal A304 A336
  constraint tangent L230 A337
  constraint tangent L231 A337
  constraint equal A304 A337
  constraint tangent L228 A338
  constraint tangent L231 A338
  constraint equal A304 A338
  constraint tangent L228 A339
  constraint tangent L229 A339
  constraint equal A304 A339
  constraint tangent L233 A340
  constraint tangent L234 A340
  constraint equal A304 A340
  constraint tangent L234 A341
  constraint tangent L235 A341
  constraint equal A304 A341
  constraint tangent L232 A342
  constraint tangent L235 A342
  constraint equal A304 A342
  constraint tangent L232 A343
  constraint tangent L233 A343
  constraint equal A304 A343
  constraint tangent L237 A344
  constraint tangent L238 A344
  constraint equal A304 A344
  constraint tangent L238 A345
  constraint tangent L239 A345
  constraint equal A304 A345
  constraint tangent L236 A346
  constraint tangent L239 A346
  constraint equal A304 A346
  constraint tangent L236 A347
  constraint tangent L237 A347
  constraint equal A304 A347
  constraint tangent L241 A348
  constraint tangent L242 A348
  constraint equal A304 A348
  constraint tangent L242 A349
  constraint tangent L243 A349
  constraint equal A304 A349
  constraint tangent L240 A350
  constraint tangent L241 A350
  constraint equal A304 A350
  constraint tangent L240 A351
  constraint tangent L243 A351
  constraint equal A304 A351
  constraint tangent L245 A352
  constraint tangent L246 A352
  constraint equal A304 A352
  constraint tangent L244 A353
  constraint tangent L245 A353
  constraint equal A304 A353
  constraint tangent L244 A354
  constraint tangent L247 A354
  constraint equal A304 A354
  constraint tangent L246 A355
  constraint tangent L247 A355
  constraint equal A304 A355
  constraint tangent L50 A356
  constraint tangent L51 A356
  constraint equal A304 A356
  constraint tangent L48 A357
  constraint tangent L51 A357
  constraint equal A304 A357
  constraint tangent L48 A358
  constraint tangent L49 A358
  constraint equal A304 A358
  constraint tangent L49 A359
  constraint tangent L50 A359
  constraint equal A304 A359
  constraint tangent L52 A360
  constraint tangent L55 A360
  constraint equal A304 A360
  constraint tangent L54 A361
  constraint tangent L55 A361
  constraint equal A304 A361
  constraint tangent L53 A362
  constraint tangent L54 A362
  constraint equal A304 A362
  constraint tangent L52 A363
  constraint tangent L53 A363
  constraint equal A304 A363
  constraint tangent L57 A364
  constraint tangent L59 A364
  constraint equal A304 A364
  constraint tangent L56 A365
  constraint tangent L57 A365
  constraint equal A304 A365
  constraint tangent L56 A366
  constraint tangent L58 A366
  constraint equal A304 A366
  constraint tangent L58 A367
  constraint tangent L59 A367
  constraint equal A304 A367
  constraint tangent L61 A368
  constraint tangent L63 A368
  constraint equal A304 A368
  constraint tangent L60 A369
  constraint tangent L61 A369
  constraint equal A304 A369
  constraint tangent L60 A370
  constraint tangent L62 A370
  constraint equal A304 A370
  constraint tangent L62 A371
  constraint tangent L63 A371
  constraint equal A304 A371
  constraint tangent L65 A372
  constraint tangent L67 A372
  constraint equal A304 A372
  constraint tangent L64 A373
  constraint tangent L65 A373
  constraint equal A304 A373
  constraint tangent L64 A374
  constraint tangent L66 A374
  constraint equal A304 A374
  constraint tangent L66 A375
  constraint tangent L67 A375
  constraint equal A304 A375
  constraint tangent L69 A376
  constraint tangent L71 A376
  constraint equal A304 A376
  constraint tangent L68 A377
  constraint tangent L69 A377
  constraint equal A304 A377
  constraint tangent L68 A378
  constraint tangent L70 A378
  constraint equal A304 A378
  constraint tangent L70 A379
  constraint tangent L71 A379
  constraint equal A304 A379
  constraint tangent L73 A380
  constraint tangent L75 A380
  constraint equal A304 A380
  constraint tangent L72 A381
  constraint tangent L73 A381
  constraint equal A304 A381
  constraint tangent L72 A382
  constraint tangent L74 A382
  constraint equal A304 A382
  constraint tangent L74 A383
  constraint tangent L75 A383
  constraint equal A304 A383
  constraint tangent L77 A384
  constraint tangent L79 A384
  constraint equal A304 A384
  constraint tangent L76 A385
  constraint tangent L77 A385
  constraint equal A304 A385
  constraint tangent L76 A386
  constraint tangent L78 A386
  constraint equal A304 A386
  constraint tangent L78 A387
  constraint tangent L79 A387
  constraint equal A304 A387
  constraint tangent L81 A388
  constraint tangent L83 A388
  constraint equal A304 A388
  constraint tangent L80 A389
  constraint tangent L81 A389
  constraint equal A304 A389
  constraint tangent L80 A390
  constraint tangent L82 A390
  constraint equal A304 A390
  constraint tangent L82 A391
  constraint tangent L83 A391
  constraint equal A304 A391
  constraint tangent L85 A392
  constraint tangent L87 A392
  constraint equal A304 A392
  constraint tangent L84 A393
  constraint tangent L85 A393
  constraint equal A304 A393
  constraint tangent L84 A394
  constraint tangent L86 A394
  constraint equal A304 A394
  constraint tangent L86 A395
  constraint tangent L87 A395
  constraint equal A304 A395
  constraint tangent L89 A396
  constraint tangent L91 A396